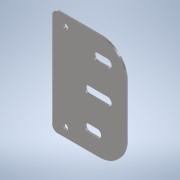
# Autodesk Inventor part: adjust_sheet
Saved by Autodesk Inventor 2021 (Build 250183000, 183)
## iProperties
Created: 2021-06-23
Part Number: adjust_sheet
Material: Steel, Mild
Document SubType Name: Modeling
Density: 7.85 g/cm^3
Appearance: Semi-Polished
Mass: 361.224 g
Surface Area: 329.393 cm^2
Volume: 46.0158 cm^3
Autodesk Inventor part; units mm, degrees
ref_plane "YZ Plane" through (0, 0, 0) normal (1, 0, 0) x (0, 1, 0)
ref_plane "XZ Plane" through (0, 0, 0) normal (0, 1, 0) x (-1, 0, 0)
ref_plane "XY Plane" through (0, 0, 0) normal (0, 0, 1) x (1, 0, 0)
sketch "Sketch1" plane through (0, 0, 0) normal (0, 0, 1) x (1, 0, 0)
  circle A0 centre (1008.2886, -225.2) radius 1095
  line L0 (-27.5, 131.7988) -> (-27.5, 31.7988)
  line L1 (-43.3188, 130) -> (-43.3188, 30)
  line L2 (-56.5579, 30) -> (-56.5579, 130)
  line L3 (-27.5, 130) -> (-56.5579, 130)
  line L4 (-27.5, 80) -> (-56.5579, 80)
  line L5 (-27.5, 30) -> (-56.5579, 30)
  line L6 (-111.5579, 160) -> (0, 160)
  line L7 (0, 160) -> (0, 0)
  line L8 (0, 0) -> (-111.5579, 0)
  line L9 (-111.5579, 0) -> (-111.5579, 160)
  point P0 (0, 0)
  point P1 (-43.3188, 80)
  dimension "d4" = 2190
  dimension "d10" = 50
  dimension "d11" = 50
  dimension "d21" = 305.2
  dimension "d36" = 30
  dimension "d37" = 30
  dimension "d38" = 27.5
  dimension "d39" = 55
  constraints: 26 end point, 8 point on line, 4 horizontal, 4 parallel, 3 point on circle, 3 vertical, 2 coincident, 2 midpoint, 1 centre point, 1 perpendicular
  measures "d4" diameter of A0
  measures "d10" distance between parallel lines of L3 L4
  measures "d11" distance between parallel lines of L5 L4
  measures "d21" vertical distance of A0.centre A0.end
  measures "d36" distance from line of L6 L3.start
  measures "d37" distance from line of L8 point (-43.319, 30)
  measures "d38" distance from line of L7 L3.start
  measures "d39" distance from line of L9 point (-56.558, 80)
extrude "Extrusion1" add sketch "Sketch1" along normal blind 3 contours L6 L7 L8 A0 L5 L1 L4 L0 | A0 L3 L2 L8 L9 L6 | L0 L4 A0 | A0 L1 L3 | L2 L4 A0 | A0 L1 L5 | L4 L2 L3 L1
hole "Hole1" at (-27.5, 130, 0) at (-43.3188, 80, 0) at (-56.5579, 30, 0) at (-43.3188, 130, 0) at (-27.5, 80, 0) at (-43.3188, 30, 0) at (-56.5579, 80, 0) direction (0, 0, 1) diameter 12 end through all
sketch "Sketch2" plane through (0, 0, 0) normal (0, 0, -1) x (-1, 0, 0)
  circle A0 centre (27.5, 130) radius 6 projected
  circle A1 centre (43.3188, 130) radius 6 projected
  line L0 (27.5, 124) -> (43.3188, 124)
  circle A2 centre (27.5, 130) radius 6 projected
  line L1 (27.5, 136) -> (43.3188, 136)
  line L2 (27.5, 136) -> (27.5, 124)
  line L3 (43.3188, 124) -> (43.3188, 136)
  line L4 (27.5, 86) -> (56.5579, 86)
  line L5 (27.5, 74) -> (56.5579, 74)
  circle A3 centre (27.5, 80) radius 6 projected
  circle A4 centre (56.5579, 80) radius 6 projected
  line L6 (27.5, 86) -> (27.5, 74)
  line L7 (56.5579, 74) -> (56.5579, 86)
  line L8 (43.3188, 36) -> (56.5579, 36)
  line L9 (43.3188, 24) -> (56.5579, 24)
  circle A5 centre (43.3188, 30) radius 6 projected
  circle A6 centre (56.5579, 30) radius 6 projected
  line L10 (43.3188, 24) -> (43.3188, 36)
  line L11 (56.5579, 24) -> (56.5579, 36)
  point P0 (0, 0)
  constraints: 24 end point, 10 point on circle, 8 horizontal, 4 tangent, 3 parallel, 3 vertical, 1 vertical alignment, 3 other
extrude "Extrusion2" cut sketch "Sketch2" against normal blind 3 contours A0 L1 A1 L0 | L4 A4 L5 A3 | L8 A6 L9 A5
sketch "Sketch3" plane through (0, 0, 3) normal (0, 0, 1) x (1, 0, 0)
  line L0 (-111.5579, 160) -> (-111.5579, 0) projected
  line L1 (0, 160) -> (-111.5579, 160) projected
  line L2 (-111.5579, 0) -> (0, 0) projected
  line L3 (-56.5579, 86) -> (-27.5, 86) projected
  line L4 (-27.5, 124) -> (-43.3188, 124) projected
  line L5 (-27.5, 74) -> (-56.5579, 74) projected
  line L6 (-56.5579, 36) -> (-43.3188, 36) projected
  point P0 (-91.5579, 146)
  point P1 (-91.5579, 14)
  dimension "d51" = 20
  dimension "d52" = 14
  dimension "d53" = 14
  dimension "d54" = 20
  measures "d51" distance from line of L0 point (-91.558, 14)
  measures "d52" distance from line of L2 point (-91.558, 14)
  measures "d53" distance from line of L1 point (-91.558, 146)
  measures "d54" distance from line of L0 point (-91.558, 146)
hole "Hole2" at (-91.5579, 14, 3) at (-91.5579, 146, 3) direction (0, 0, -1) diameter 8 end through all
fillet "Fillet2" radius 40 2 edges at (0, 0, 1.5) (0, 160, 1.5)
fillet "Fillet3" radius 8 2 edges at (-111.5579, 0, 1.5) (-111.5579, 160, 1.5)
equation "\"d11\" = d10"
equation "\"d37\" = d36"
equation "\"d39\" = 2 * d38"
body "Solid1"
